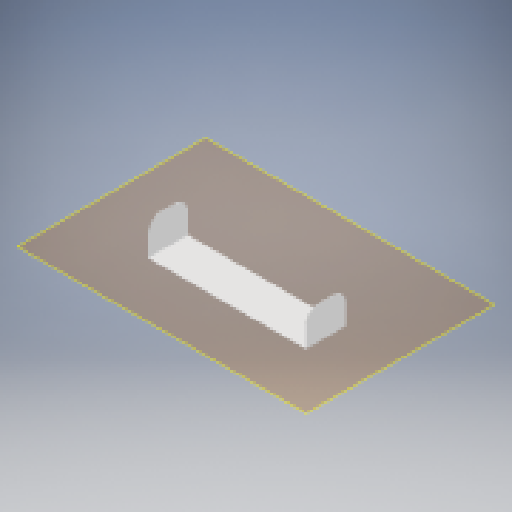
# Autodesk Inventor part: CE-5.2.3-03
Saved by Autodesk Inventor 2024 (Build 280153000, 153)
## iProperties
Created: 2024-02-15
Part Number: CE-5.2.3-03
Material: Generic
Document SubType Name: Sheet Metal
Designer: Alex
Density: 1 g/cm^3
Sheet Metal Rule: Default
Appearance: Default
Author: Alex
Autodesk Inventor part; units mm, degrees
ref_plane "YZ Plane" through (0, 0, 0) normal (1, 0, 0) x (0, 1, 0)
ref_plane "XZ Plane" through (0, 0, 0) normal (0, 1, 0) x (-1, 0, 0)
ref_plane "XY Plane" through (0, 0, 0) normal (0, 0, 1) x (1, 0, 0)
ref_plane "Work Plane1" through (-420.2595, 673.9641, 1040.2284) normal (0, 1, 0) x (-1, 0, 0)
sketch "Sketch1" plane through (-420.2595, 673.9641, 1040.2284) normal (0, 1, 0) x (-1, 0, 0)
  line L0 (-1974.87, 175.87) -> (-25.13, 175.87) construction
  line L1 (-25.13, -175.87) -> (-1974.87, -175.87) construction
  line L2 (-24.13, 0) -> (-24.13, 224.13) construction
  line L3 (-1975.87, -224.13) -> (-1975.87, 0) construction
  line L4 (-1975.87, 0) -> (-1975.87, 224.13) construction
  line L5 (-24.13, -224.13) -> (-24.13, 0) construction
  line L6 (-300, 175.87) -> (-1700, 175.87)
  line L7 (-1700, 175.87) -> (-1700, -175.87)
  line L8 (-1700, -175.87) -> (-300, -175.87)
  line L9 (-300, -175.87) -> (-300, 175.87)
  point P0 (-420.2595, -1040.2284)
  point P1 (-1000, 175.87)
  point P2 (-1000, -175.87)
  point P3 (-1000, -175.87)
  dimension "d0" = 1400
  measures "d0" distance between parallel lines of L7 L9
extrude "Plate1" add sketch "Sketch1" along normal blind 3.048
sketch "Sketch2" plane through (1276.6925, 673.9641, 864.3584) normal (1, 0, 0) x (0, 1, 0)
  line L0 (0, 351.74) -> (0, 0)
  line L1 (0, 0) -> (300, 0)
  line L2 (300, 0) -> (300, 351.74)
  line L3 (300, 351.74) -> (0, 351.74)
  constraints: 6 end point, 1 horizontal, 1 perpendicular, 1 vertical
edge flange "Flange1" height 300 angle 90 thickness 3.048 bend radius 3.048 thickness toward (1, 0, 0) relief tear relief width 3.048 relief depth 1.524 corner gap 3.048 corner form 0 edges at (1279.7405, 677.0121, 1040.2284) (-120.2595, 677.0121, 1040.2284) wall of the first edge with corners at (1276.6925, 673.9641, 1216.0984) (1276.6925, 673.9641, 864.3584) (1276.6925, 973.9641, 864.3584) (1276.6925, 973.9641, 1216.0984)
bend "Bend1"
corner "Corner1"
fillet "Corner Round1" radius 120 4 edges at (-118.7355, 973.9641, 1216.0984) (-118.7355, 973.9641, 864.3584) (1278.2165, 973.9641, 1216.0984) (1278.2165, 973.9641, 864.3584)
equation "\"d1\" = Thickness"
equation "\"d2\" = BendReliefWidth"
equation "\"d3\" = BendReliefDepth"
equation "\"d4\" = MinimumRemnant"
equation "\"d5\" = TransitionRadius"
equation "\"d8\" = BendRadius"
equation "\"d9\" = CornerReliefSize"
equation "\"d10\" = GapSize"
equation "\"d11\" = JacobiRadiusSize"
equation "\"BendRadius\" = Thickness"
equation "\"BendReliefWidth\" = Thickness"
equation "\"BendReliefDepth\" = 0.5 * Thickness"
equation "\"CornerReliefSize\" = 4 * Thickness"
equation "\"MinimumRemnant\" = 2 * Thickness"
equation "\"TransitionRadius\" = BendRadius"
equation "\"JacobiRadiusSize\" = BendRadius"
equation "\"GapSize\" = Thickness"
equation "\"Thickness\" = 3.048"
body "Solid1"
